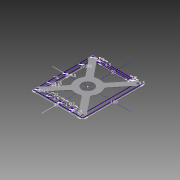
# Autodesk Inventor part: Side
Saved by Autodesk Inventor 2014 SP1 (Build 180222100, 222)
## iProperties
Created: 2015-03-28
Part Number: Side
Material: Generic
Document SubType Name: Modeling
Designer: Erin
Density: 1 g/cm^3
Appearance: Default
Author: Erin
Autodesk Inventor part; units mm, degrees
ref_plane "YZ Plane" through (0, 0, 0) normal (1, 0, 0) x (0, 1, 0)
ref_plane "XZ Plane" through (0, 0, 0) normal (0, 1, 0) x (-1, 0, 0)
ref_plane "XY Plane" through (0, 0, 0) normal (0, 0, 1) x (1, 0, 0)
sketch "Sketch1" plane through (0, 0, 0) normal (0, 0, 1) x (1, 0, 0)
  line L0 (-41.5, 50) -> (41.5, 50)
  line L1 (41.5, 50) -> (41.5, -50)
  line L2 (41.5, -50) -> (-41.5, -50)
  line L3 (-41.5, -50) -> (-41.5, 50)
  line L4 (35.5, 44) -> (-35.5, 44)
  line L5 (-35.5, 44) -> (-35.5, -44)
  line L6 (-35.5, -44) -> (35.5, -44)
  line L7 (35.5, -44) -> (35.5, 44)
  line L8 (-41.5, -47) -> (41.5, -47) construction
  circle A0 centre (-19.75, -47) radius 2.25
  line L9 (0, 71.7466) -> (0, -78.0681) construction
  circle A1 centre (0, -47) radius 2.25
  circle A2 centre (19.75, -47) radius 2.25
  line L10 (-60.2597, 0) -> (74.2823, 0) construction
  line L11 (-38.5, 50) -> (-38.5, -50) construction
  circle A3 centre (-38.5, 0) radius 2.25
  circle A4 centre (-38.5, 27) radius 2.25
  circle A5 centre (-38.5, -27) radius 2.25
  line L12 (-41.5, 47) -> (41.5, 47) construction
  line L13 (-35.5, -3) -> (-35.5, 3)
  circle A6 centre (-38.5, 47) radius 2.25
  circle A7 centre (-38.5, -47) radius 2.25
  line L14 (-25, 50) -> (25, 50)
  line L15 (25, 50) -> (25, 47)
  line L16 (25, 47) -> (-25, 47)
  line L17 (-25, 47) -> (-25, 50)
  circle A8 centre (-28, 47) radius 2.25
  circle A9 centre (28, 47) radius 2.25
  point P0 (0, 0)
  point P1 (0, 50)
  point P2 (41.5, 0)
  point P3 (0, 47)
  point P4 (0, 47)
  dimension "d0" = 83
  dimension "d1" = 100
  dimension "d2" = 4.5
  dimension "d3" = 4.5
  dimension "d4" = 4.5
  dimension "d5" = 3
  dimension "d6" = 3
  dimension "d9" = 3
  dimension "d10" = 4.5
  dimension "d11" = 4.5
  dimension "d12" = 4.5
  dimension "d17" = 3
  dimension "d41" = 4.5
  dimension "d42" = 4.5
  dimension "d45" = 29.25
  dimension "d46" = 29.25
  dimension "d47" = 22
  dimension "d48" = 22
  dimension "d66" = 50
  dimension "d67" = 3
  dimension "d81" = 4.5
  dimension "d82" = 4.5
  dimension "d83" = 3
  dimension "d84" = 3
  constraints: 36 end point, 19 point on line, 10 centre point, 8 perpendicular, 6 midpoint, 6 parallel, 3 horizontal, 2 vertical alignment, 1 horizontal alignment, 1 vertical, 3 other
  measures "d0" distance of L1.end L2.end
  measures "d1" distance of L0.end L1.end
  measures "d2" diameter of A0
  measures "d3" diameter of A1
  measures "d4" diameter of A2
  measures "d5" distance between parallel lines of L8 L2
  measures "d6" distance between parallel lines of L6 L8
  measures "d9" distance between parallel lines of L11 L3
  measures "d10" diameter of A3
  measures "d11" diameter of A4
  measures "d12" diameter of A5
  measures "d17" distance between parallel lines of L12 L0
  measures "d41" diameter of A6
  measures "d42" diameter of A7
  measures "d66" distance of L15.end L16.end
  measures "d67" distance of L14.end L15.end
  measures "d81" diameter of A8
  measures "d82" diameter of A9
  measures "d83" distance from line of A8.centre L17
  measures "d84" distance from line of A9.centre L15
sketch "Sketch5" plane through (0, 0, 0) normal (0, 0, 1) x (1, 0, 0)
  circle A0 centre (-28, 47) radius 2.25
  circle A1 centre (28, 47) radius 2.25
  circle A2 centre (38.5, 47) radius 2.25
  circle A3 centre (38.5, 27) radius 2.25
  circle A4 centre (38.5, 0) radius 2.25
  circle A5 centre (38.5, -27) radius 2.25
  circle A6 centre (38.5, -47) radius 2.25
  circle A7 centre (-38.5, 47) radius 2.25
  circle A8 centre (-38.5, 27) radius 2.25
  circle A9 centre (-38.5, 0) radius 2.25
  circle A10 centre (-38.5, -27) radius 2.25
  circle A11 centre (-38.5, -47) radius 2.25
  line L0 (35.5, 44) -> (35.5, -44)
  line L1 (35.5, -44) -> (-35.5, -44)
  line L2 (-35.5, -44) -> (-35.5, 44)
  line L3 (-35.5, 44) -> (35.5, 44)
  circle A12 centre (19.75, -47) radius 2.25
  circle A13 centre (0, -47) radius 2.25
  circle A14 centre (-19.75, -47) radius 2.25
  line L4 (-41.5, 50) -> (-41.5, -50)
  line L5 (-41.5, -50) -> (41.5, -50)
  line L6 (41.5, -50) -> (41.5, 50)
  line L7 (41.5, 50) -> (-41.5, 50)
  circle A15 centre (0, 0) radius 10
  circle A16 centre (0, 0) radius 20
  line L8 (-4.2057, -2.75) -> (-40.0923, 41.7291)
  line L9 (-40.0923, 41.7291) -> (-32.3095, 48.0083)
  line L10 (-32.3095, 48.0083) -> (3.577, 3.5292)
  line L11 (3.577, 3.5292) -> (-4.2057, -2.75)
  line L12 (0, 0) -> (-35.5, 44) construction
  line L13 (-0.3143, 0.3896) -> (-36.2009, 44.8687) construction
  line L14 (-41.5, 50) -> (-31.5, 50)
  line L15 (-31.5, 50) -> (-31.5, 40)
  line L16 (-31.5, 40) -> (-41.5, 40)
  line L17 (-41.5, 40) -> (-41.5, 50)
  point P0 (0, 0)
  point P1 (0, 0.3896)
  dimension "d87" = 20
  dimension "d88" = 10
  dimension "d89" = 10
  dimension "d98" = 10
  dimension "d99" = 10
  constraints: 36 end point, 17 centre point, 4 parallel, 3 coincident, 2 midpoint, 2 perpendicular, 1 collinear, 1 horizontal, 1 horizontal alignment
  measures "d87" diameter of A15
  measures "d88" radial gap between concentric circles of A15 A16
  measures "d89" distance of L8.end L9.end
  measures "d98" distance of L15.end L16.end
  measures "d99" distance of L14.end L15.end
extrude "Extrusion8" add sketch "Sketch5" along normal blind 0.6 contours L10 A16 L8 L2 L16 L15 L3 | L3 L15 L10 | L15 L16 L2 L3 | L3 L2 L16 L8 L9 L10 L15 | L10 L9 L8 L16 L4 L7 L15 | L10 A15 L8 A16 | A16 L8 A15 L10 | L8 L16 L2
extrude "Extrusion9" cut sketch "Sketch5" along normal blind 10 contours L10 L11 L8 A15 | A15 L8 L11 L10
fillet "Fillet1" radius 3 2 edges at (-16.0511, 11.9316, 0.3) (-8.2684, 18.2108, 0.3)
mirror "Mirror2" about plane through (0, 0, 0) normal (1, 0, 0) of "Extrusion8", "Extrusion9", "Fillet1"
mirror "Mirror3" about plane through (0, 0, 0) normal (0, 1, 0) of "Extrusion8", "Extrusion9", "Fillet1", "Mirror2"
fillet "Fillet3" radius 2 4 edges at (-41.5, 40, 0.3) (-38.6972, 40, 0.3) (-31.5, 47.005, 0.3) (-31.5, 50, 0.3)
mirror "Mirror4" about plane through (0, 0, 0) normal (1, 0, 0) of "Fillet3"
mirror "Mirror5" about plane through (0, 0, 0) normal (0, 1, 0) of "Fillet3", "Mirror4"
body "Solid1"
